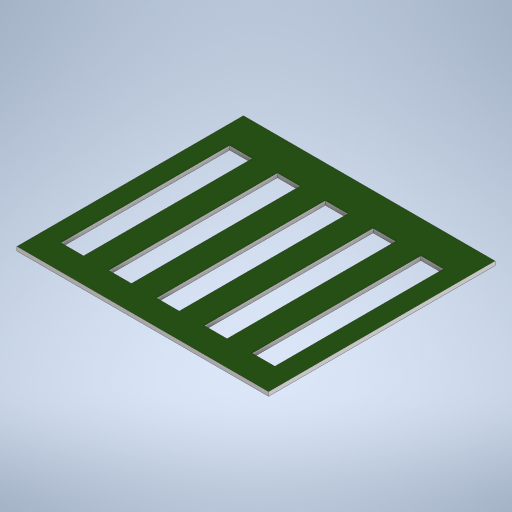
# Autodesk Inventor part: TopPCB
Saved by Autodesk Inventor 2023 (Build 270158000, 158)
## iProperties
Created: 2024-03-19
Part Number: TopPCB
Material: Generic
Document SubType Name: Modeling
Designer: noname
Density: 1 g/cm^3
Appearance: Default
Author: noname
Autodesk Inventor part; units mm, degrees
ref_plane "YZ Plane" through (0, 0, 0) normal (1, 0, 0) x (0, 1, 0)
ref_plane "XZ Plane" through (0, 0, 0) normal (0, 1, 0) x (-1, 0, 0)
ref_plane "XY Plane" through (0, 0, 0) normal (0, 0, 1) x (1, 0, 0)
sketch "Sketch1" plane through (0, 0, 0) normal (0, 1, 0) x (-1, 0, 0)
  line L0 (0, 0) -> (-100, 0)
  line L1 (-100, 0) -> (-100, -90)
  line L2 (-100, -90) -> (0, -90)
  line L3 (0, -90) -> (0, 0)
  line L4 (-10.5, -77) -> (-13.5, -77)
  line L5 (-13.5, -77) -> (-13.5, -10)
  line L6 (-13.5, -10) -> (-10.5, -10)
  line L7 (-10.5, -10) -> (-10.5, -77)
  line L8 (-29.5, -77) -> (-32.5, -77)
  line L9 (-32.5, -77) -> (-32.5, -10)
  line L10 (-32.5, -10) -> (-29.5, -10)
  line L11 (-29.5, -10) -> (-29.5, -77)
  line L12 (-48.5, -77) -> (-51.5, -77)
  line L13 (-51.5, -77) -> (-51.5, -10)
  line L14 (-51.5, -10) -> (-48.5, -10)
  line L15 (-48.5, -10) -> (-48.5, -77)
  line L16 (-67.5, -77) -> (-70.5, -77)
  line L17 (-70.5, -77) -> (-70.5, -10)
  line L18 (-70.5, -10) -> (-67.5, -10)
  line L19 (-67.5, -10) -> (-67.5, -77)
  line L20 (-86.5, -77) -> (-89.5, -77)
  line L21 (-89.5, -77) -> (-89.5, -10)
  line L22 (-89.5, -10) -> (-86.5, -10)
  line L23 (-86.5, -10) -> (-86.5, -77)
  point P0 (-10.5, -43.5)
  point P1 (-29.5, -43.5)
  point P2 (-48.5, -43.5)
  point P3 (-67.5, -43.5)
  point P4 (-86.5, -43.5)
  dimension "d1" = 90
  dimension "d2" = 3
  dimension "d3" = 67
  dimension "d4" = 10.5
  dimension "d7" = 19
  dimension "d12" = 10.5
  dimension "d26" = 10
  constraints: 48 end point, 4 parallel, 3 horizontal, 2 perpendicular, 1 midpoint, 36 other
  measures "d1" distance between parallel lines of L0 L2
  measures "d2" distance between parallel lines of L5 L7
  measures "d3" distance between parallel lines of L4 L6
  measures "d4" distance between parallel lines of L3 L7
  measures "d7" distance of L4.start L8.start
  measures "d12" distance between parallel lines of L1 L21
  measures "d26" distance between parallel lines of L0 L6
extrude "Extrusion1" add sketch "Sketch1" along normal blind 1.6
sketch "Sketch2" plane through (0, 1.6, 0) normal (0, 1, 0) x (1, 0, 0)
  line L0 (100, 0) -> (100, 90) projected
  line L1 (100, 90) -> (0, 90) projected
  line L2 (0, 90) -> (0, 0) projected
  line L3 (0, 0) -> (100, 0) projected
  line L4 (86.5, 77) -> (89.5, 77) projected
  line L5 (89.5, 77) -> (89.5, 10) projected
  line L6 (89.5, 10) -> (86.5, 10) projected
  line L7 (86.5, 10) -> (86.5, 77) projected
  line L8 (67.5, 77) -> (70.5, 77) projected
  line L9 (70.5, 77) -> (70.5, 10) projected
  line L10 (70.5, 10) -> (67.5, 10) projected
  line L11 (67.5, 10) -> (67.5, 77) projected
  line L12 (48.5, 77) -> (51.5, 77) projected
  line L13 (51.5, 77) -> (51.5, 10) projected
  line L14 (51.5, 10) -> (48.5, 10) projected
  line L15 (48.5, 10) -> (48.5, 77) projected
  line L16 (29.5, 77) -> (32.5, 77) projected
  line L17 (32.5, 77) -> (32.5, 10) projected
  line L18 (32.5, 10) -> (29.5, 10) projected
  line L19 (29.5, 10) -> (29.5, 77) projected
  line L20 (10.5, 77) -> (13.5, 77) projected
  line L21 (13.5, 77) -> (13.5, 10) projected
  line L22 (13.5, 10) -> (10.5, 10) projected
  line L23 (10.5, 10) -> (10.5, 77) projected
  line L24 (7.5, 10) -> (16.5, 10)
  line L25 (16.5, 10) -> (16.5, 77)
  line L26 (16.5, 77) -> (7.5, 77)
  line L27 (7.5, 77) -> (7.5, 10)
  line L28 (35.5, 10) -> (35.5, 77)
  line L29 (26.5, 10) -> (35.5, 10)
  line L30 (26.5, 77) -> (26.5, 10)
  line L31 (35.5, 77) -> (26.5, 77)
  line L32 (54.5, 10) -> (54.5, 77)
  line L33 (45.5, 10) -> (54.5, 10)
  line L34 (45.5, 77) -> (45.5, 10)
  line L35 (54.5, 77) -> (45.5, 77)
  line L36 (73.5, 10) -> (73.5, 77)
  line L37 (64.5, 10) -> (73.5, 10)
  line L38 (64.5, 77) -> (64.5, 10)
  line L39 (73.5, 77) -> (64.5, 77)
  line L40 (92.5, 10) -> (92.5, 77)
  line L41 (83.5, 10) -> (92.5, 10)
  line L42 (83.5, 77) -> (83.5, 10)
  line L43 (92.5, 77) -> (83.5, 77)
  point P0 (12, 77)
  point P1 (12, 10)
  point P2 (31, 10)
  point P3 (31, 77)
  point P4 (50, 10)
  point P5 (50, 77)
  point P6 (69, 10)
  point P7 (69, 77)
  point P8 (88, 10)
  point P9 (88, 77)
  dimension "d15" = 9
  dimension "d18" = 19
  constraints: 40 end point, 4 midpoint, 2 horizontal, 2 parallel, 1 perpendicular, 40 other
  measures "d15" distance between parallel lines of L25 L27
  measures "d18" distance of L24.end L28.start
extrude "Extrusion2" cut sketch "Sketch2" against normal blind 10 contours L4 L5 L6 L7 | L7 L41 L42 L43 | L43 L40 L41 L5 | L8 L9 L10 L11 | L11 L37 L38 L39 | L39 L36 L37 L9 | L12 L13 L14 L15 | L15 L33 L34 L35 | L35 L32 L33 L13 | L16 L17 L18 L19 | L19 L29 L30 L31 | L31 L28 L29 L17 | L20 L21 L22 L23 | L23 L24 L27 L26 | L26 L25 L24 L21
body "Solid1"
